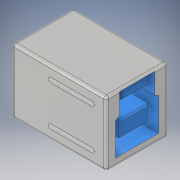
# Autodesk Inventor part: USB_halter
Saved by Autodesk Inventor 2017 (Build 210142000, 142)
## iProperties
Part Number: USB_halter
Material: Generisch
Document SubType Name: Modeling
Designer: ExCISS
Density: 1 g/cm^3
Appearance: Vorgabe
Author: ExCISS
Autodesk Inventor part; units mm, degrees
ref_plane "YZ Plane" through (0, 0, 0) normal (1, 0, 0) x (0, 1, 0)
ref_plane "XZ Plane" through (0, 0, 0) normal (0, 1, 0) x (-1, 0, 0)
ref_plane "XY Plane" through (0, 0, 0) normal (0, 0, 1) x (1, 0, 0)
sketch "Skizze2" plane through (0, 0, 0) normal (0, 0, 1) x (1, 0, 0)
  line L0 (-9.225, 6.025) -> (9.225, 6.025)
  line L1 (9.225, 6.025) -> (9.225, -6.025)
  line L2 (9.225, -6.025) -> (-9.225, -6.025)
  line L3 (-9.225, -6.025) -> (-9.225, 6.025)
  line L4 (-9.225, 6.025) -> (9.225, -6.025) construction
  point P0 (0, 0)
  point P1 (0, 0)
  dimension "d0" = 18.45
  dimension "d1" = 12.05
  constraints: 10 end point, 2 parallel, 1 coincident, 1 horizontal, 1 midpoint, 1 perpendicular
  measures "d0" distance of L1.end L2.end
  measures "d1" distance of L0.end L1.end
extrude "Extrusion1" add sketch "Skizze2" along normal blind 12.67
sketch "Skizze3" plane through (9.225, -6.025, 0) normal (1, 0, 0) x (0, 0, -1)
  line L0 (-1.53, 1.77) -> (-1.53, 10.28)
  line L1 (-1.53, 10.28) -> (-7.88, 10.28)
  line L2 (-1.53, 1.77) -> (-7.88, 1.77)
  line L3 (0, 6.025) -> (-1.53, 6.025)
  line L4 (0, 6.025) -> (1.53, 6.025) construction
  line L5 (0, 12.05) -> (-12.67, 12.05) construction
  line L6 (-12.67, 12.05) -> (-12.37, 12.05) construction
  line L7 (-12.37, 12.05) -> (-12.37, 9.47) construction
  line L8 (-12.37, 9.47) -> (-8.37, 9.47)
  line L9 (-12.37, 9.47) -> (-8.37, 9.47) construction
  line L10 (-8.37, 9.47) -> (-7.88, 10.28)
  line L11 (-12.67, 12.05) -> (-12.67, 0) construction
  line L12 (-12.67, 0) -> (-12.37, 0) construction
  line L13 (0, 0) -> (-12.67, 0) construction
  line L14 (-12.37, 0) -> (-12.37, 2.58) construction
  line L15 (-12.37, 2.58) -> (-8.37, 2.58)
  line L16 (-8.37, 2.58) -> (-7.88, 1.77)
  line L17 (-12.37, 2.58) -> (-12.37, 9.47)
  dimension "d4" = 8.51
  dimension "d5" = 6.35
  dimension "d6" = 6.35
  dimension "d7" = 1.53
  dimension "d8" = 180
  dimension "d9" = 0.3
  dimension "d10" = 2.58
  dimension "d11" = 4
  dimension "d13" = 0.3
  dimension "d14" = 2.58
  dimension "d15" = 4
  constraints: 30 end point, 6 horizontal, 3 perpendicular, 2 collinear, 2 point on line, 1 midpoint, 1 vertical
  measures "d4" distance of L0.start L0.end
  measures "d5" distance of L0.end L1.end
  measures "d6" distance of L0.start L2.end
  measures "d7" distance of L3.end L3.start
  measures "d8" angle of L3 L4
  measures "d9" distance of L5.end L6.end
  measures "d10" distance of L6.end L7.end
  measures "d11" distance of L7.end L8.end
  measures "d13" distance of L11.end L12.end
  measures "d14" distance of L12.end L14.end
  measures "d15" distance of L14.end L15.end
extrude "Extrusion2" cut sketch "Skizze3" against normal blind 8.88
fillet "Rundung1" radius 0.5 12 edges at (0, -6.025, 12.67) (0, -6.025, 0) (0, 6.025, 12.67) (0, 6.025, 0) (9.225, 0, 0) (9.225, 0, 12.67) (-9.225, -6.025, 6.335) (-9.225, 0, 12.67) (-9.225, 6.025, 6.335) (-9.225, 0, 0) (9.225, -6.025, 6.335) (9.225, 6.025, 6.335)
sketch "Skizze4" plane through (0.345, -6.025, 0) normal (1, 0, 0) x (0, 0, -1)
  line L0 (-1.53, 10.28) -> (-1.53, 1.77) construction
  line L1 (-7.88, 10.28) -> (-1.53, 10.28) construction
  line L2 (-8.37, 9.47) -> (-7.88, 10.28) construction
  line L3 (-12.37, 9.47) -> (-8.37, 9.47) construction
  line L4 (-12.37, 2.58) -> (-12.37, 9.47) construction
  line L5 (-8.37, 2.58) -> (-12.37, 2.58) construction
  line L6 (-7.88, 1.77) -> (-8.37, 2.58) construction
  line L7 (-1.53, 1.77) -> (-7.88, 1.77) construction
  line L8 (-1.53, 1.77) -> (-7.88, 1.77) construction
  line L9 (-1.53, 1.77) -> (-3.85, 1.77) construction
  line L10 (-3.85, 1.77) -> (-3.85, 3.18) construction
  line L11 (-3.85, 3.18) -> (-1.53, 3.18) construction
  line L12 (-1.53, 3.18) -> (-1.53, 1.77) construction
  line L13 (-3.85, 3.18) -> (-7, 3.18)
  line L14 (-7, 3.18) -> (-7, 8.8)
  line L15 (-7, 8.8) -> (-3.85, 8.8)
  line L16 (-3.85, 8.8) -> (-3.85, 3.18)
  point P0 (0, 6.025)
  dimension "d19" = 2.32
  dimension "d20" = 1.41
  dimension "d21" = 3.15
  dimension "d22" = 5.62
  constraints: 16 end point, 4 parallel, 2 horizontal, 2 perpendicular
  measures "d19" distance of L10.end L11.end
  measures "d20" distance of L9.end L10.end
  measures "d21" distance of L14.end L15.end
  measures "d22" distance of L13.end L14.end
extrude "Extrusion3" add sketch "Skizze4" along normal blind 8.4
chamfer "Fase1" distance 0.3 angle 45 4 edges at (8.745, -0.035, 7) (8.745, -2.845, 5.425) (8.745, -0.035, 3.85) (8.745, 2.775, 5.425)
sketch "Skizze5" plane through (0.345, -6.025, 0) normal (1, 0, 0) x (0, 0, -1)
  line L0 (-12.37, 2.58) -> (-12.37, 9.47) projected
  line L1 (-12.37, 9.47) -> (-11.47, 9.47)
  line L2 (-11.47, 9.47) -> (-11.47, 8.63) construction
  line L3 (-11.47, 8.63) -> (-12.37, 8.63) construction
  line L4 (-12.37, 8.63) -> (-12.37, 9.47)
  line L5 (-12.37, 2.58) -> (-11.47, 2.58) construction
  line L6 (-11.47, 2.58) -> (-11.47, 3.42) construction
  line L7 (-11.47, 3.42) -> (-12.37, 3.42) construction
  line L8 (-12.37, 3.42) -> (-12.37, 2.58) construction
  line L9 (-7, 8.8) -> (-7, 3.18) construction
  line L10 (-7, 5.99) -> (-10.32, 5.99) construction
  line L11 (-11.47, 3.42) -> (-10.32, 3.42)
  line L12 (-10.32, 3.42) -> (-10.32, 8.63)
  line L13 (-10.32, 8.63) -> (-11.47, 8.63)
  line L14 (-11.47, 8.63) -> (-11.47, 3.42)
  point P0 (0, 6.025)
  dimension "d28" = 0.9
  dimension "d29" = 0.84
  dimension "d30" = 0.9
  dimension "d31" = 0.84
  dimension "d32" = 3.32
  constraints: 26 end point, 6 parallel, 4 horizontal, 3 perpendicular, 1 midpoint
  measures "d28" distance of L2.end L3.end
  measures "d29" distance of L1.end L2.end
  measures "d30" distance of L7.end L6.end
  measures "d31" distance of L6.end L5.end
  measures "d32" distance of L10.start L10.end
extrude "Extrusion4" add sketch "Skizze5" along normal blind 8.4
chamfer "Fase2" distance 0.1 angle 45 4 edges at (8.745, 2.605, 10.895) (8.745, 0, 11.47) (8.745, -2.605, 10.895) (8.745, 0, 10.32)
sketch "Skizze6" plane through (-8.725, -6.025, 0.5) normal (0, -1, 0) x (1, 0, 0)
  line L0 (6.6009, 1.8619) -> (15.6009, 1.8619) construction
  line L1 (7.0761, 2.3371) -> (15.1257, 2.3371)
  line L2 (15.1257, 1.3867) -> (7.0761, 1.3867)
  arc A0 (7.0761, 2.3371) -> (7.0761, 1.3867) centre (7.0761, 1.8619) ccw
  arc A1 (15.1257, 1.3867) -> (15.1257, 2.3371) centre (15.1257, 1.8619) ccw
  line L3 (6.6009, 9.7163) -> (15.6009, 9.7163) construction
  line L4 (7.0761, 10.1915) -> (15.1257, 10.1915)
  line L5 (15.1257, 9.2411) -> (7.0761, 9.2411)
  arc A2 (7.0761, 10.1915) -> (7.0761, 9.2411) centre (7.0761, 9.7163) ccw
  arc A3 (15.1257, 9.2411) -> (15.1257, 10.1915) centre (15.1257, 9.7163) ccw
  point P0 (8.725, -0.5)
  point P1 (11.1009, 1.8619)
  point P2 (11.1009, 9.7163)
  dimension "d38" = 9
  dimension "d39" = 9
  constraints: 16 end point, 12 point on circle, 8 tangent, 4 centre point, 4 point on line, 2 horizontal, 2 midpoint, 2 parallel
  measures "d38" distance of L0.start L0.end
  measures "d39" distance of L3.start L3.end
extrude "Extrusion7" cut sketch "Skizze6" against normal blind 0.01
sketch "Skizze7" plane through (-8.725, 6.025, 0.5) normal (0, 1, 0) x (1, 0, 0)
  line L0 (6.563, -9.7202) -> (15.563, -9.7202) construction
  line L1 (7.0382, -9.2451) -> (15.0878, -9.2451)
  line L2 (15.0878, -10.1954) -> (7.0382, -10.1954)
  arc A0 (7.0382, -9.2451) -> (7.0382, -10.1954) centre (7.0382, -9.7202) ccw
  arc A1 (15.0878, -10.1954) -> (15.0878, -9.2451) centre (15.0878, -9.7202) ccw
  line L3 (6.563, -1.8658) -> (15.563, -1.8658) construction
  line L4 (7.0382, -1.3907) -> (15.0878, -1.3907)
  line L5 (15.0878, -2.341) -> (7.0382, -2.341)
  arc A2 (7.0382, -1.3907) -> (7.0382, -2.341) centre (7.0382, -1.8658) ccw
  arc A3 (15.0878, -2.341) -> (15.0878, -1.3907) centre (15.0878, -1.8658) ccw
  line L6 (17.45, -11.67) -> (17.45, 0) construction
  line L7 (17.45, -11.67) -> (15.126, -11.67) construction
  line L8 (15.126, -11.67) -> (15.126, -10.192) construction
  line L9 (15.126, -10.192) -> (17.45, -10.192) construction
  line L10 (17.45, -10.192) -> (17.45, -11.67) construction
  point P0 (8.725, 0.5)
  point P1 (8.725, -0.5)
  point P2 (11.063, -9.7202)
  point P3 (11.063, -1.8658)
  dimension "d46" = 9
  dimension "d47" = 9
  dimension "d48" = 2.324
  dimension "d49" = 1.478
  constraints: 24 end point, 12 point on circle, 8 tangent, 4 centre point, 4 parallel, 4 point on line, 3 horizontal, 2 midpoint, 1 perpendicular
  measures "d46" distance of L0.start L0.end
  measures "d47" distance of L3.start L3.end
  measures "d48" distance of L8.end L9.end
  measures "d49" distance of L7.end L8.end
extrude "Extrusion8" cut sketch "Skizze7" against normal blind 0.01
